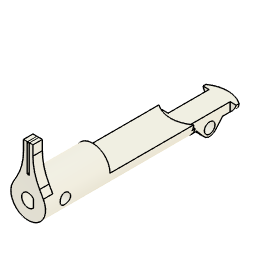
marker_motor_coupling_new (Autodesk Fusion 360 archive; units mm, degrees)
design "marker_motor_coupling_new" references "NEMA17 42-40"
Autodesk Fusion 360 part; units mm, degrees
derive "Esquisse1" from "NEMA17 42-40 v4"
sketch "Esquisse1" plane through (0, 0, 0) normal (0, 1, 0) x (-1, 0, 0)
  line L0 (-1.945, 1.5707) -> (-1.945, -1.5707) construction
  arc A0 (-1.945, -1.5707) -> (-1.945, 1.5707) centre (0, 0) ccw construction
  arc A1 (-2.095, -1.6228) -> (-2.095, 1.6228) centre (0, 0) ccw
  line L1 (-2.095, 1.6228) -> (-2.095, -1.6228)
  dimension "d35" = 0.15
sketch "Esquisse3" plane through (0, 0, 0) normal (1, 0, 0) x (0, 1, 0)
  line L0 (0, 7) -> (20, 7)
  line L1 (20, 25) -> (23, 25)
  line L2 (0, 0) -> (23, 0)
  line L3 (23, 25) -> (23, 0)
  line L4 (0, 0) -> (0, 7)
  line L5 (20, 7) -> (20, 25)
  point P0 (0, -11)
  point P1 (0, 7)
  point P2 (23, 25)
  point P3 (23, 0)
  dimension "d19" = 3
  dimension "d22" = 25
  dimension "d33" = 7
  dimension "d37" = 23
  constraint coincident P1 L0.start
  constraint horizontal L0
  constraint coincident P2 L1.end
  constraint coincident L2.start L4.start
  constraint horizontal L2
  constraint coincident P3 L2.end
  constraint vertical L5
  constraint horizontal L1
  constraint vertical L3
  constraint coincident L0.end L5.start
  constraint vertical L4
  measures "d19" distance of L1.start P2
  measures "d22" distance of L1 L2
  measures "d33" distance of P1 L2.start
  measures "d37" distance of L3 L4
revolve "Révolution1" add sketch "Esquisse3" angle 360 about axis through (0, 0, 0) along (0, 1, 0)
extrude "Extrusion3" cut sketch "Esquisse1" along normal through all
sketch "Esquisse4" plane through (0, 20, 0) normal (0, -1, 0) x (1, 0, 0)
  circle A0 centre (0, 0) radius 25
  line L0 (0, 0) -> (0, 22)
  circle A1 centre (0, 0) radius 7
  dimension "d23" = 22
  constraint coincident A0.centre L0.start
  constraint vertical L0
  measures "d23" distance of A0.centre L0.end
ref_plane "Plan de construction2" through (7, 3.3841, 0) normal (1, 0, 0) x (0, 0, 1)
sketch "Esquisse6" plane through (7, 0, 0) normal (1, 0, 0) x (0, 1, 0)
  line L0 (0, 1.6228) -> (0, -1.6228)
  line L1 (0, -7) -> (0, 7)
  line L2 (20, -7) -> (20, 7)
  line L3 (0, 0) -> (8, 0) construction
  dimension "d41" = 8
  constraint coincident L3.start origin
  constraint perpendicular L1 L3
  measures "d41" distance of L3.start L3.end
hole "Perçage3" at (7, 8, 0) direction (-1, 0, 0) diameter 3.2 end up to surface (7 mm away) counterbore diameter 4.2 counterbore depth 4.2
delete_face "DeleteFace1" 1 faces at (0, 20, -18.9511)
sketch "Esboço7" plane through (0, 23, 0) normal (0, 1, 0) x (-1, 0, 0)
  line L0 (-2.095, -1.6228) -> (-2.095, 1.6228)
  arc A0 (-2.095, -1.6228) -> (-2.095, 1.6228) centre (0, 0) ccw
  circle A1 centre (0, 0) radius 7
  line L1 (0, 0) -> (7, 0)
  line L2 (0, 0) -> (-7, 0)
  arc A2 (-7, 0) -> (7, 0) centre (0, 0) ccw
  constraint coincident A0.centre A1.centre
  constraint coincident A1 L1.end
  constraint horizontal L1
  constraint coincident A1 L2.end
  constraint parallel L1 L2
extrude "Extrusão4" add sketch "Esboço7" along normal blind 57.5 contours L0 A0 A1 L1 L2 A2 | L0 A0 L1 L2 picked at (-1.3967, -0.5409)
ref_plane "Plano de trabalho3" through (0, 69, 3.5) normal (0, 1, 0) x (0, 0, 1)
sketch "Esboço11" plane through (0, 0, 0) normal (0, 0, 1) x (-1, 0, 0)
  line L0 (7, -23) -> (2.65, -23)
  line L1 (2.65, -23) -> (-2.095, -23)
  line L2 (-2.095, -23) -> (-7, -23)
  line L3 (-7, -23) -> (-7, -80.5)
  line L4 (-7, -80.5) -> (7, -80.5)
  line L5 (7, -80.5) -> (7, -23)
  circle A0 centre (-0.0034, -68.95) radius 11.55
  line L6 (-10.7789, -73.1081) -> (-10.7789, -83.552)
  line L7 (-10.7789, -83.552) -> (11.6456, -83.552)
  line L8 (11.6456, -83.552) -> (11.5464, -68.8719)
  dimension "d71" = 23.1
  constraint tangent L4 A0
  constraint coincident A0 L6.start
  constraint vertical L6
  constraint perpendicular L6 L7
  constraint coincident A0 L8.end
  constraint tangent A0 L8
  measures "d71" diameter of A0
extrude "Extrusão7" cut sketch "Esboço11" against normal blind 2 contours L5 A0 L8 | L3 L5 A0 | L3 A0
extrude "Extrusão8" cut 4 faces at (-6.5503, 79.2186, 0) (-2.3585, 80.3511, 0) (6.626, 79.178, 0) (1.864, 80.408, 0) along direction (0, 0, -1) blind 17
sketch "Esboço12" plane through (0, 0, -2) normal (0, 0, 1) x (-1, 0, 0)
  line L0 (-6.7082, -59.5453) -> (-6.7082, -78.3547)
  arc A0 (-6.7082, -78.3547) -> (6.7082, -78.3499) centre (-0.0034, -68.95) ccw
  line L1 (6.7082, -78.3499) -> (6.7082, -59.5501)
  arc A1 (6.7082, -59.5501) -> (-6.7082, -59.5453) centre (-0.0034, -68.95) ccw
  line L2 (-4.2534, -77.2) -> (4.2466, -77.2)
  line L3 (4.2466, -77.2) -> (4.2466, -60.7)
  line L4 (4.2466, -60.7) -> (-4.2534, -60.7)
  line L5 (-4.2534, -60.7) -> (-4.2534, -77.2)
  line L6 (-4.2534, -77.2) -> (4.2466, -60.7) construction
  line L7 (4.2466, -77.2) -> (-4.2534, -60.7) construction
  line L8 (6.7082, -77.2) -> (-6.7149, -77.2)
  line L9 (-6.7149, -77.2) -> (-6.7149, -60.7)
  line L10 (-6.7149, -60.7) -> (6.7082, -60.7)
  line L11 (6.7082, -60.7) -> (6.7082, -77.2)
  line L12 (6.7082, -77.2) -> (-6.7149, -60.7) construction
  line L13 (-6.7149, -77.2) -> (6.7082, -60.7) construction
  point P0 (-0.0034, -68.95)
  point P1 (-0.0034, -68.95)
  dimension "d76" = 8.5
  dimension "d77" = 16.5
  dimension "d87" = 16.5
  constraint horizontal L2
  constraint perpendicular L2 L3
  constraint parallel L2 L4
  constraint parallel L3 L5
  constraint coincident L6 P1
  constraint coincident L7 P1
  constraint coincident P1 P0
  constraint horizontal L8
  constraint perpendicular L8 L9
  constraint parallel L8 L10
  constraint parallel L9 L11
  constraint coincident L12 P1
  constraint coincident L13 P1
  constraint coincident L1 L8.start
  measures "d76" distance of L3.end L4.end
  measures "d77" distance of L2.end L3.end
  measures "d87" distance of L8.end L9.end
extrude "Extrusão9" cut sketch "Esboço12" against normal blind 13 contours L0 L5 L8 L10 | L0 L8 L9 L10 | L1 L3 L8 L10 L11
sketch "Esboço13" plane through (4.2534, 0, 0) normal (1, 0, 0) x (0, 1, 0)
  line L0 (60.7, -5.5596) -> (77.2, -5.5596)
  line L1 (77.2, -5.5596) -> (77.2, -2)
  line L2 (77.2, -2) -> (60.7, -2)
  line L3 (60.7, -2) -> (60.7, -5.5596)
  line L4 (66.6701, -8.9807) -> (60.7, -2)
  arc A0 (66.6701, -8.9807) -> (71.2299, -8.9807) centre (68.95, -7.0309) ccw
  line L5 (60.7, -2) -> (77.2, -2)
  line L6 (77.2, -2) -> (71.2299, -8.9807)
  circle A1 centre (68.95, -7.0309) radius 2.15
  point P0 (60.7, -2)
  dimension "d80" = 16.5
  dimension "d81" = 3
  dimension "d82" = 4.3
  constraint coincident P0 L2.end
  constraint horizontal L5
  constraint tangent L4 A0
  constraint tangent A0 L6
  constraint concentric A0 A1
  constraint midpoint L2 L5
  measures "d80" distance of L1.end P0
  measures "d81" radius of A0
  measures "d82" diameter of A1
extrude "Extrusão10" add sketch "Esboço13" against normal blind 8.524 contours L0 L4 A0 L6 A1
extrude "Extrusão11" cut sketch "Esboço13" against normal blind 39 contours L0 A1 | L0 A1
sketch "Esboço10" plane through (0, 23, 0) normal (0, 1, 0) x (-1, 0, 0)
  line L0 (-7, 0) -> (-2.095, 0)
  line L1 (-2.095, 0) -> (-2.095, 1.6228)
  arc A0 (2.65, 0) -> (-2.095, 1.6228) centre (0, 0) ccw
  line L2 (2.65, 0) -> (7, 0)
  arc A1 (7, 0) -> (-7, 0) centre (0, 0) ccw
  line L3 (-7, 0) -> (7, 0)
  arc A2 (7, 0) -> (-7, 0) centre (0, 0) ccw
  constraint coincident L0.start A1.end
  constraint coincident L2.end A1.start
  constraint coincident A0.centre A1.centre
extrude "Extrusão6" add sketch "Esboço10" along normal blind 3
sketch "Esboço16" plane through (0, 0, 0) normal (0, -1, 0) x (1, 0, 0)
  circle A0 centre (0, 0) radius 7
  line L0 (1.9, 7) -> (-1.9, 7)
  line L1 (-1.9, 16.4007) -> (-1.9, 37)
  line L2 (-1.9, 37) -> (1.9, 37)
  line L3 (1.9, 37) -> (1.9, 16.4007)
  line L4 (1.9, 7) -> (-1.9, 37) construction
  line L5 (-1.9, 7) -> (1.9, 37) construction
  line L6 (-4.598, 6.1033) -> (-6.1007, 3.4325)
  line L7 (4.598, 6.1033) -> (6.1007, 3.4325)
  arc A1 (-4.598, 6.1033) -> (-1.9, 16.4007) centre (-22.9, 16.4007) ccw
  arc A2 (1.9, 16.4007) -> (4.598, 6.1033) centre (22.9, 16.4007) ccw
  point P0 (0, 22)
  dimension "d101" = 3.8
  dimension "d102" = 30
  dimension "d103" = 21
  constraint horizontal L0
  constraint perpendicular L0 L1
  constraint parallel L0 L2
  constraint parallel L1 L3
  constraint coincident L4 P0
  constraint coincident L5 P0
  constraint tangent A0 L0
  constraint coincident A0 L6.end
  constraint tangent A0 L6
  constraint coincident A0 L7.end
  constraint tangent A0 L7
  constraint coincident L0.end L1
  constraint tangent L6 A1
  constraint tangent L1 A1
  constraint coincident L0.start L3
  constraint tangent L7 A2
  constraint tangent L3 A2
  constraint equal A1 A2
  measures "d101" distance of L1.end L2.end
  measures "d102" distance of L0.end L1.end
  measures "d103" radius of A1
extrude "Extrusão13" add sketch "Esboço16" against normal blind 3.8 contours A0 L1 L2 L3 L6 L7 A1 A2
sketch "Esboço17" plane through (0, 0, 0) normal (0, -1, 0) x (1, 0, 0)
  line L0 (2.095, 1.6228) -> (2.095, -1.6228)
  arc A0 (2.095, 1.6228) -> (2.095, -1.6228) centre (0, 0) ccw
  arc A1 (-6.1007, 3.4325) -> (6.1007, 3.4325) centre (0, 0) ccw
  line L1 (6.1007, 3.4325) -> (4.598, 6.1033)
  arc A2 (1.9, 16.4007) -> (4.598, 6.1033) centre (22.9, 16.4007) ccw
  line L2 (1.9, 16.4007) -> (1.9, 37)
  line L3 (1.9, 37) -> (-1.9, 37)
  line L4 (-1.9, 37) -> (-1.9, 16.4007)
  arc A3 (-4.598, 6.1033) -> (-1.9, 16.4007) centre (-22.9, 16.4007) ccw
  line L5 (-4.598, 6.1033) -> (-6.1007, 3.4325)
  line L6 (0.3852, 20.15) -> (-0.4148, 20.15)
  line L7 (-0.4148, 20.15) -> (-0.4148, 9)
  line L8 (-0.4148, 9) -> (0.3852, 9)
  line L9 (0.3852, 9) -> (0.3852, 20.15)
  line L10 (0.3852, 20.15) -> (-0.4148, 9) construction
  line L11 (-0.4148, 20.15) -> (0.3852, 9) construction
  line L12 (-5.1392, 20.35) -> (5.9735, 20.35)
  line L13 (5.9735, 20.35) -> (5.9735, 40.35)
  line L14 (5.9735, 40.35) -> (-5.1392, 40.35)
  line L15 (-5.1392, 40.35) -> (-5.1392, 20.35)
  point P0 (-0.0148, 14.575)
  dimension "d104" = 0.8
  dimension "d105" = 11.15
  dimension "d109" = 0.2
  dimension "d110" = 20
  constraint horizontal L6
  constraint perpendicular L6 L7
  constraint parallel L6 L8
  constraint parallel L7 L9
  constraint coincident L10 P0
  constraint coincident L11 P0
  constraint horizontal L12
  constraint vertical L13
  constraint horizontal L14
  constraint vertical L15
  measures "d104" distance of L7.end L8.end
  measures "d105" distance of L6.end L7.end
  measures "d109" distance of L6.end L12
  measures "d110" distance of L12.end L13.end
extrude "Extrusão14" cut sketch "Esboço17" against normal blind 10 contours L2 L3 L4 L12 | L6 L7 L8 L9
